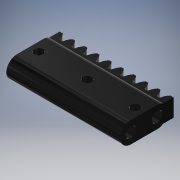
# Autodesk Inventor part: GA04
Saved by Autodesk Inventor 2017 (Build 210142000, 142)
## iProperties
Created: 2018-10-24
Part Number: GA04
Material: ABS Plastic
Document SubType Name: Modeling
Designer: Dell
Density: 1.06 g/cm^3
Appearance: Smooth - Black
Author: Dell
Autodesk Inventor part; units mm, degrees
ref_plane "YZ Plane" through (0, 0, 0) normal (1, 0, 0) x (0, 1, 0)
ref_plane "XZ Plane" through (0, 0, 0) normal (0, 1, 0) x (-1, 0, 0)
ref_plane "XY Plane" through (0, 0, 0) normal (0, 0, 1) x (1, 0, 0)
sketch "Sketch1" plane through (0, 0, 0) normal (0, 0, 1) x (1, 0, 0)
  spline S0 degree 3 poles (-2.7752, 20.8158) (-2.7042, 20.7277) (-2.562, 20.5515) (-2.36, 20.2785) (-2.1667, 19.9993) (-1.9839, 19.7131) (-1.8126, 19.4198) (-1.654, 19.1195) (-1.5101, 18.8118) (-1.3833, 18.4967) (-1.2955, 18.2274) (-1.2397, 18.008) (-1.2095, 17.8408) (-1.1935, 17.6716) (-1.162, 17.5046) (-1.1186, 17.3404) (-1.0623, 17.18) (-0.9883, 17.0268) (-0.8958, 16.884) (-0.7836, 16.7557) (-0.6724, 16.6674) (-0.5769, 16.6065) (-0.4998, 16.5707) (-0.4208, 16.5391) (-0.3383, 16.5188) (-0.2547, 16.503) (-0.1414, 16.4982) (0, 16.5012) (0.1414, 16.4982) (0.2547, 16.503) (0.3383, 16.5188) (0.4208, 16.5391) (0.4998, 16.5707) (0.5769, 16.6065) (0.6724, 16.6674) (0.7836, 16.7557) (0.8958, 16.884) (0.9883, 17.0268) (1.0623, 17.18) (1.1186, 17.3404) (1.162, 17.5046) (1.1935, 17.6716) (1.2095, 17.8408) (1.2397, 18.008) (1.2955, 18.2274) (1.3833, 18.4967) (1.5101, 18.8118) (1.654, 19.1195) (1.8126, 19.4198) (1.9839, 19.7131) (2.1667, 19.9993) (2.36, 20.2785) (2.562, 20.5515) (2.7042, 20.7277) (2.7752, 20.8158) knots 0 0 0 0 0.033953 0.067907 0.10186 0.135813 0.169766 0.203718 0.237669 0.271619 0.305565 0.322541 0.339512 0.356488 0.373464 0.390436 0.407409 0.424381 0.44135 0.458313 0.475267 0.483756 0.492243 0.500732 0.509218 0.517706 0.526192 0.543169 0.560147 0.568632 0.577121 0.585607 0.594095 0.602582 0.611072 0.628025 0.644989 0.661958 0.67893 0.695903 0.712875 0.729851 0.746827 0.763798 0.780774 0.81472 0.84867 0.882621 0.916573 0.950526 0.984479 1.018432 1.052385 1.086339 1.086339 1.086339 1.086339
  circle A0 centre (0, 0) radius 16.5 construction
  circle A1 centre (0, 0) radius 17.8542 construction
  circle A2 centre (0, 0) radius 19 construction
  circle A3 centre (0, 0) radius 21 construction
  line L0 (-2.7752, 20.8158) -> (2.7752, 20.8158)
  point P0 (-2.5639, 20.5501)
  point P1 (-2.3614, 20.2775)
  point P2 (-2.1684, 19.9981)
  point P3 (-1.9858, 19.7119)
  point P4 (-1.8147, 19.4186)
  point P5 (-1.6565, 19.1183)
  point P6 (-1.513, 18.8106)
  point P7 (-1.3869, 18.4953)
  point P8 (-1.2828, 18.1722)
  point P9 (-1.2417, 18.0075)
  point P10 (-1.2119, 17.8405)
  point P11 (-1.1909, 17.672)
  point P12 (-1.16, 17.5051)
  point P13 (-1.1164, 17.341)
  point P14 (-1.0594, 17.1812)
  point P15 (-0.9852, 17.0285)
  point P16 (-0.8925, 16.8864)
  point P17 (-0.78, 16.7594)
  point P18 (-0.648, 16.653)
  point P19 (-0.576, 16.6082)
  point P20 (-0.4995, 16.5714)
  point P21 (-0.4202, 16.541)
  point P22 (-0.3381, 16.5195)
  point P23 (-0.2545, 16.505)
  point P24 (-0.1698, 16.5)
  point P25 (0, 16.5)
  point P26 (0.1698, 16.5)
  point P27 (0.2545, 16.505)
  point P28 (0.3381, 16.5195)
  point P29 (0.4202, 16.541)
  point P30 (0.4995, 16.5714)
  point P31 (0.576, 16.6082)
  point P32 (0.648, 16.653)
  point P33 (0.78, 16.7594)
  point P34 (0.8925, 16.8864)
  point P35 (0.9852, 17.0285)
  point P36 (1.0594, 17.1812)
  point P37 (1.1164, 17.341)
  point P38 (1.16, 17.5051)
  point P39 (1.1909, 17.672)
  point P40 (1.2119, 17.8405)
  point P41 (1.2417, 18.0075)
  point P42 (1.2828, 18.1722)
  point P43 (1.3869, 18.4953)
  point P44 (1.513, 18.8106)
  point P45 (1.6565, 19.1183)
  point P46 (1.8147, 19.4186)
  point P47 (1.9858, 19.7119)
  point P48 (2.1684, 19.9981)
  point P49 (2.3614, 20.2775)
  point P50 (2.5639, 20.5501)
  constraints: 4 centre point, 2 end point, 2 point on circle, 1 horizontal, 111 other
sketch "Sketch2" plane through (0, 0, 0) normal (0, 0, 1) x (1, 0, 0)
  line L0 (32.5, 20.8158) -> (-32.5, 20.8158)
  line L1 (-32.5, 20.8158) -> (-32.5, 14.8158)
  line L2 (-32.5, 14.8158) -> (32.5, 14.8158)
  line L3 (32.5, 14.8158) -> (32.5, 20.8158)
  circle A0 centre (0, 0) radius 21 construction
  point P0 (0, 20.8158)
  point P1 (-2.7752, 20.8158)
  point P2 (2.7752, 20.8158)
  dimension "d2" = 6
  dimension "d3" = 65
  constraints: 8 end point, 2 parallel, 1 horizontal, 1 midpoint, 1 perpendicular, 1 point on line, 1 vertical alignment
  measures "d2" distance of L0.end L1.end
  measures "d3" distance of L1.end L2.end
extrude "Extrusion2" add sketch "Sketch2" along normal blind 10
extrude "Extrusion3" cut sketch "Sketch1" along normal blind 10
pattern_linear "Rectangular Pattern1" count 9 spacing 6.9446 along (-1, 0, 0) of "Extrusion3" first direction both ways yes
sketch "Sketch3" plane through (-32.5, 14.8158, 0) normal (-1, 0, 0) x (0, 0, 1)
  circle A0 centre (5, -3.3166) radius 6
  line L0 (0, 0) -> (10, 0) projected
  point P0 (0, -14.8158)
  point P1 (5, 0)
  dimension "d11" = 12
  constraints: 2 point on circle, 1 centre point, 1 midpoint, 1 vertical alignment
  measures "d11" diameter of A0
extrude "Extrusion4" add sketch "Sketch3" against normal blind 65 contours A0 L0 picked at (5.1596, -3.0992)
sketch "Sketch6" plane through (32.5, 20.8158, 10) normal (1, 0, 0) x (0, 0, -1)
  circle A0 centre (5, -24.3166) radius 6
  arc A1 (0, -6) -> (10, -6) centre (5, -9.3166) ccw projected
  line L0 (-1, -24.3166) -> (-1, -9.3166)
  line L1 (11, -9.3166) -> (11, -24.3166)
  arc A2 (-1, -9.3166) -> (11, -9.3166) centre (5, -9.3166) ccw
  point P0 (10, -20.8158)
  dimension "d21" = 15
  dimension "d22" = 12
  constraints: 6 point on circle, 4 end point, 4 tangent, 2 centre point, 1 concentric, 1 vertical alignment
  measures "d21" distance of A1.centre A0.centre
  measures "d22" diameter of A0
extrude "Extrusion6" add sketch "Sketch6" against normal blind 65
sketch "Sketch7" plane through (32.5, 20.8158, 10) normal (1, 0, 0) x (0, 0, -1)
  arc A0 (-1, -24.3166) -> (11, -24.3166) centre (5, -24.3166) ccw projected
  arc A1 (0, -6) -> (-1, -9.3166) centre (5, -9.3166) ccw projected
  circle A2 centre (5, -24.3166) radius 3
  circle A3 centre (5, -9.3166) radius 3
  point P0 (10, -20.8158)
  dimension "d25" = 6
  dimension "d26" = 6
  constraints: 2 centre point, 2 coincident
  measures "d25" diameter of A2
  measures "d26" diameter of A3
extrude "Extrusion7" cut sketch "Sketch7" against normal through all
sketch "Sketch8" plane through (32.5, -3.5008, 11) normal (0, 0, 1) x (1, 0, 0)
  line L0 (-65, 12) -> (-65, 18) projected
  line L1 (0, 18) -> (0, 12) projected
  line L2 (-65, -3) -> (-65, 3) projected
  line L3 (0, 3) -> (0, -3) projected
  circle A0 centre (-60, 7.5) radius 2.5
  circle A1 centre (-5, 7.5) radius 2.5
  circle A2 centre (-32.5, 7.5) radius 2.5
  line L4 (-5, 7.5) -> (-60, 7.5) construction
  line L5 (0, -6) -> (-65, -6) projected
  line L6 (-65, 3) -> (-65, 12)
  point P0 (-32.5, 3.5008)
  point P1 (-32.5, -6)
  point P2 (-65, 7.5)
  dimension "d29" = 5
  dimension "d30" = 5
  dimension "d31" = 5
  dimension "d32" = 55
  constraints: 4 end point, 3 centre point, 3 midpoint, 1 coincident, 1 horizontal, 1 horizontal alignment, 1 vertical, 1 vertical alignment
  measures "d29" diameter of A0
  measures "d30" diameter of A1
  measures "d31" diameter of A2
  measures "d32" distance of L4.start L4.end
extrude "Extrusion8" cut sketch "Sketch8" against normal through all
equation "\"Module\" = 2"
equation "\"PressureAngle\" = 20deg"
equation "\"UnitProfileClearance\" = 0.25"
equation "\"UnitRoundRadius\" = 0.35"
equation "\"HeadDiameter\" = 42"
equation "\"RootDiameter\" = 33"
equation "\"BaseDiameter\" = 35.70832"
equation "\"PitchDiameter\" = 38"
equation "\"HelixAngle\" = 0"
equation "\"UnitCorrection\" = 0"
equation "\"UnitAddendumModification\" = 0"
equation "\"CircularPitch\" = 6.283185"
equation "\"UnitBacklashShift\" = 0"
equation "\"TotalToolShift\" = 0"
equation "\"IsInternal\" = 0"
body "Solid2"
